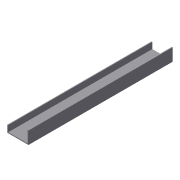
# Autodesk Inventor part: FrameFandB
Saved by Autodesk Inventor 2015 (Build 190159000, 159)
## iProperties
Created: 2015-03-05
Part Number: FrameFandB
Material: Generic
Document SubType Name: Modeling
Designer: Kyle
Density: 1 g/cm^3
Appearance: Default
Author: Kyle
Autodesk Inventor part; units mm, degrees
ref_plane "YZ Plane" through (0, 0, 0) normal (1, 0, 0) x (0, 1, 0)
ref_plane "XZ Plane" through (0, 0, 0) normal (0, 1, 0) x (-1, 0, 0)
ref_plane "XY Plane" through (0, 0, 0) normal (0, 0, 1) x (1, 0, 0)
sketch "Sketch1" plane through (0, 0, 0) normal (0, 0, 1) x (1, 0, 0)
  line L0 (0, 0) -> (85.725, 0)
  line L1 (0, 0) -> (85.725, 0) construction
  line L2 (85.725, 0) -> (85.725, 50.8)
  line L3 (85.725, 50.8) -> (82.55, 50.8)
  line L4 (82.55, 50.8) -> (82.55, 3.175)
  line L5 (82.55, 3.175) -> (3.175, 3.175)
  line L6 (3.175, 3.175) -> (3.175, 28.575)
  line L7 (3.175, 28.575) -> (0, 28.575)
  line L8 (0, 28.575) -> (0, 0)
  dimension "d0" = 85.725
  dimension "d1" = 0
  dimension "d2" = 50.8
  dimension "d3" = 90
  dimension "d4" = 3.175
  dimension "d5" = 47.625
  dimension "d6" = 79.375
  dimension "d7" = 25.4
  constraints: 18 end point, 5 perpendicular, 2 horizontal, 1 collinear, 1 parallel, 1 vertical
  measures "d0" distance of L0.start L0.end
  measures "d1" distance between parallel lines of L0 L1
  measures "d2" distance of L0.end L2.end
  measures "d3" angle of L2 L0
  measures "d4" distance of L2.end L3.end
  measures "d5" distance of L3.end L4.end
  measures "d6" distance of L4.end L5.end
  measures "d7" distance of L5.end L6.end
extrude "Extrusion1" add sketch "Sketch1" along normal blind 584.2
body "Solid1"
